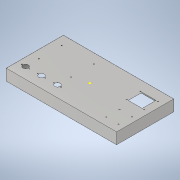
# Autodesk Inventor part: Gehaeuse_Deckel
Saved by Autodesk Inventor 2020 (Build 240168000, 168)
## iProperties
Created: 2019-01-15
Part Number: Gehaeuse_Deckel
Material: Generic
Document SubType Name: Modeling
Designer: patri
Density: 1 g/cm^3
Appearance: Aluminum - Polished
Author: Patrik Staudenmayer
Autodesk Inventor part; units mm, degrees
ref_plane "YZ Plane" through (0, 0, 0) normal (1, 0, 0) x (0, 1, 0)
ref_plane "XZ Plane" through (0, 0, 0) normal (0, 1, 0) x (-1, 0, 0)
ref_plane "XY Plane" through (0, 0, 0) normal (0, 0, 1) x (1, 0, 0)
sketch "Sketch1" plane through (0, 0, 0) normal (0, 1, 0) x (-1, 0, 0)
  line L0 (222, -115) -> (-222, -115)
  line L1 (-222, -115) -> (-222, 115)
  line L2 (-222, 115) -> (222, 115)
  line L3 (222, 115) -> (222, -115)
  line L4 (0, -161) -> (0, 161) projected
  line L5 (310.8, 0) -> (-310.8, 0) projected
  point P0 (0, 0)
  dimension "d0" = 444
  dimension "d1" = 230
  constraints: 8 end point, 2 parallel, 1 horizontal, 1 perpendicular, 2 other
  measures "d0" distance of L0.start L0.end
  measures "d1" distance of L0.end L1.end
extrude "Extrusion1" add sketch "Sketch1" along normal blind 45
sketch "Sketch10" plane through (0, 0, 0) normal (0, -1, 0) x (1, 0, 0)
  line L0 (-221.88, 114.88) -> (221.88, 114.88)
  line L1 (221.88, 114.88) -> (221.88, -114.88)
  line L2 (221.88, -114.88) -> (-221.88, -114.88)
  line L3 (-221.88, -114.88) -> (-221.88, 114.88)
  line L4 (0, -161) -> (0, 161) projected
  line L5 (-310.8, 0) -> (310.8, 0) projected
  line L6 (-222, 115) -> (-222, -115) projected
  line L7 (222, 115) -> (-222, 115) projected
  point P0 (0, 0)
  dimension "d19" = 0.12
  dimension "d20" = 0.12
  constraints: 8 end point, 2 parallel, 1 horizontal, 1 perpendicular, 2 other
  measures "d19" distance between parallel lines of L3 L6
  measures "d20" distance between parallel lines of L0 L7
extrude "Extrusion6" cut sketch "Sketch10" against normal blind 44.88 contours L0 L4 L5 L3 | L0 L1 L5 L4 | L5 L4 L2 L3 | L5 L1 L2 L4
sketch "Sketch11" plane through (0, 45, 0) normal (0, 1, 0) x (1, 0, 0)
  circle A0 centre (-189, -70) radius 11
  line L0 (-222, 115) -> (-222, -115) projected
  line L1 (-222, -115) -> (222, -115) projected
  circle A1 centre (-125, -70) radius 11
  circle A2 centre (-61, -70) radius 11
  line L2 (-221.88, 114.88) -> (-221.88, -114.88) projected
  line L3 (-221.88, -70) -> (1.88, -70) construction
  circle A3 centre (-174, -70) radius 2
  circle A4 centre (-204, -70) radius 2
  circle A5 centre (-140, -70) radius 2
  circle A6 centre (-110, -70) radius 2
  circle A7 centre (-76, -70) radius 2
  circle A8 centre (-46, -70) radius 2
  line L4 (-60.23, 75.55) -> (-189.48, 75.55) construction
  line L5 (-189.48, 75.55) -> (-189.48, -16.15) construction
  line L6 (-189.48, -16.15) -> (-60.23, -16.15) construction
  line L7 (-60.23, -16.15) -> (-60.23, 75.55) construction
  line L8 (222, 115) -> (-222, 115) projected
  circle A9 centre (-189.48, 75.55) radius 2
  circle A10 centre (-60.23, 75.55) radius 2
  circle A11 centre (-60.23, -16.15) radius 2
  circle A12 centre (-189.48, -16.15) radius 2
  point P0 (0, 0)
  dimension "d24" = 22
  dimension "d25" = 33
  dimension "d27" = 22
  dimension "d30" = 64
  dimension "d31" = 22
  dimension "d33" = 64
  dimension "d35" = 45
  dimension "d36" = 4
  dimension "d37" = 15
  dimension "d38" = 4
  dimension "d39" = 15
  dimension "d40" = 4
  dimension "d41" = 4
  dimension "d42" = 4
  dimension "d43" = 4
  dimension "d44" = 15
  dimension "d45" = 15
  dimension "d46" = 15
  dimension "d47" = 15
  dimension "d50" = 129.25
  dimension "d52" = 39.45
  dimension "d54" = 32.4
  dimension "d55" = 91.7
  dimension "d56" = 4
  dimension "d57" = 4
  dimension "d58" = 4
  dimension "d59" = 4
  constraints: 13 centre point, 8 end point, 4 coincident, 2 horizontal, 2 parallel, 1 perpendicular, 1 point on line, 12 other
  measures "d24" diameter of A0
  measures "d25" distance from line of L0 A0.centre
  measures "d27" diameter of A1
  measures "d30" distance of A0.centre A1.centre
  measures "d31" diameter of A2
  measures "d33" distance of A1.centre A2.centre
  measures "d36" diameter of A3
  measures "d37" distance of A0.centre A3.centre
  measures "d38" diameter of A4
  measures "d39" distance of A0.centre A4.centre
  measures "d40" diameter of A5
  measures "d41" diameter of A6
  measures "d42" diameter of A7
  measures "d43" diameter of A8
  measures "d44" distance of A5.centre A1.centre
  measures "d45" distance of A1.centre A6.centre
  measures "d46" distance of A2.centre A7.centre
  measures "d47" distance of A8.centre A2.centre
  measures "d50" distance of L4.start L4.end
  measures "d52" distance between parallel lines of L8 L4
  measures "d54" distance between parallel lines of L2 L5
  measures "d55" distance of L6.end L4.start
  measures "d56" diameter of A9
  measures "d57" diameter of A10
  measures "d58" diameter of A11
  measures "d59" diameter of A12
extrude "Extrusion7" cut sketch "Sketch11" against normal up to next
sketch "Sketch12" plane through (0, 45, 0) normal (0, 1, 0) x (1, 0, 0)
  line L0 (129, 74.35) -> (199.5, 74.35) construction
  line L1 (199.5, 74.35) -> (199.5, 18.35) construction
  line L2 (199.5, 18.35) -> (129, 18.35) construction
  line L3 (129, 18.35) -> (129, 74.35) construction
  line L4 (222, 115) -> (-222, 115) projected
  line L5 (199.5, 115) -> (199.5, -115) construction
  line L6 (-222, -115) -> (222, -115) projected
  line L7 (222, -115) -> (222, 115) projected
  circle A0 centre (129, 74.35) radius 2.1
  circle A1 centre (199.5, 74.35) radius 2.1
  circle A2 centre (199.5, 18.35) radius 2.1
  circle A3 centre (129, 18.35) radius 2.1
  point P0 (0, 0)
  dimension "d65" = 22.5
  dimension "d66" = 40.65
  dimension "d67" = 56
  dimension "d68" = 4.2
  dimension "d69" = 4.2
  dimension "d70" = 4.2
  dimension "d71" = 4.2
  dimension "d72" = 70.5
  constraints: 10 end point, 4 centre point, 4 coincident, 3 parallel, 3 point on line, 1 horizontal, 1 perpendicular, 1 vertical
  measures "d65" distance between parallel lines of L7 L5
  measures "d66" distance between parallel lines of L4 L0
  measures "d67" distance of L2.end L0.start
  measures "d68" diameter of A0
  measures "d69" diameter of A1
  measures "d70" diameter of A2
  measures "d71" diameter of A3
  measures "d72" distance of L0.start L0.end
extrude "Extrusion8" cut sketch "Sketch12" against normal up to next
sketch "Sketch13" plane through (0, 45, 0) normal (0, 1, 0) x (1, 0, 0)
  line L0 (149.8, -31.1) -> (199.5, -31.1) construction
  line L1 (199.5, -31.1) -> (199.5, -84.5) construction
  line L2 (199.5, -84.5) -> (149.8, -84.5) construction
  line L3 (149.8, -84.5) -> (149.8, -31.1) construction
  line L4 (222, -115) -> (222, 115) projected
  line L5 (-222, -115) -> (222, -115) projected
  line L6 (199.5, 74.35) -> (199.5, 18.35) construction
  line L7 (199.5, 115) -> (199.5, -115) construction
  circle A0 centre (199.5, -31.1) radius 2.1
  circle A1 centre (149.8, -31.1) radius 2.1
  circle A2 centre (149.8, -84.5) radius 2.1
  circle A3 centre (199.5, -84.5) radius 2.1
  point P0 (0, 0)
  dimension "d75" = 49.7
  dimension "d77" = 53.4
  dimension "d79" = 30.5
  dimension "d80" = 4.2
  dimension "d81" = 4.2
  dimension "d82" = 4.2
  dimension "d83" = 4.2
  constraints: 8 end point, 4 centre point, 4 coincident, 2 parallel, 1 horizontal, 1 perpendicular, 1 point on line
  measures "d75" distance of L0.start L0.end
  measures "d77" distance of L2.end L0.start
  measures "d79" distance between parallel lines of L5 L2
  measures "d80" diameter of A0
  measures "d81" diameter of A1
  measures "d82" diameter of A2
  measures "d83" diameter of A3
extrude "Extrusion9" cut sketch "Sketch13" against normal up to next
sketch "Sketch14" plane through (0, 45, 0) normal (0, 1, 0) x (1, 0, 0)
  line L0 (199.5, 74.35) -> (199.5, 18.35) construction
  line L1 (129, 74.35) -> (199.5, 74.35) construction
  line L2 (199.5, 18.35) -> (129, 18.35) construction
  line L3 (129, 18.35) -> (129, 74.35) construction
  line L4 (135.6, 74.35) -> (191.6, 74.35)
  line L5 (191.6, 74.35) -> (191.6, 18.35)
  line L6 (191.6, 18.35) -> (135.6, 18.35)
  line L7 (135.6, 18.35) -> (135.6, 74.35)
  line L8 (121.9, 81.45) -> (206.6, 81.45) construction
  line L9 (206.6, 81.45) -> (206.6, 11.25) construction
  line L10 (206.6, 11.25) -> (121.9, 11.25) construction
  line L11 (121.9, 11.25) -> (121.9, 81.45) construction
  point P0 (0, 0)
  dimension "d86" = 56
  dimension "d87" = 56
  dimension "d88" = 7.1
  dimension "d89" = 7.1
  dimension "d90" = 7.1
  dimension "d92" = 15
  dimension "d94" = 7.1
  constraints: 16 end point, 4 parallel, 2 horizontal, 2 perpendicular, 1 point on line
  measures "d86" distance of L4.start L4.end
  measures "d87" distance of L6.end L4.start
  measures "d88" distance between parallel lines of L8 L1
  measures "d89" distance between parallel lines of L10 L2
  measures "d90" distance between parallel lines of L9 L0
  measures "d92" distance between parallel lines of L9 L5
  measures "d94" distance between parallel lines of L11 L3
extrude "Extrusion10" cut sketch "Sketch14" against normal up to next
sketch "Sketch15" plane through (0, 45, 0) normal (0, 1, 0) x (1, 0, 0)
  point P0 (0, 0)
equation "\"d60\" = d56"
equation "\"d95\" = d56"
body "Solid1"
